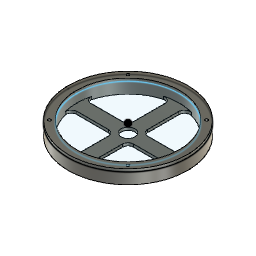
wing_interface_v1 (Autodesk Fusion 360 archive; units mm, degrees)
design "main_body_43mm_diameter"
Autodesk Fusion 360 part; units mm, degrees
(part 1 of 9)
sketch "Sketch1" plane through (0, 0, 0) normal (0, 0, 1) x (1, 0, 0)
  circle A0 centre (0, 0) radius 21.5
  circle A1 centre (0, 0) radius 18.5
  circle A2 centre (0, 0) radius 2.5
  line L0 (-2.5, 4.5) -> (-2.5, 15.8622)
  line L1 (2.5, 15.8622) -> (2.5, 4.5)
  line L2 (4.5, -2.5) -> (15.8806, -2.5)
  line L3 (15.8806, 2.5) -> (4.5, 2.5)
  line L4 (-2.5, -4.5) -> (-2.5, -15.8473)
  line L5 (2.5, -15.8473) -> (2.5, -4.5)
  line L6 (-4.5, -2.5) -> (-15.892, -2.5)
  line L7 (-15.9057, 2.5) -> (-4.5, 2.5)
  arc A3 (2.5, 4.5) -> (4.5, 2.5) centre (4.5, 4.5) ccw
  arc A4 (4.5, -2.5) -> (2.5, -4.5) centre (4.5, -4.5) ccw
  arc A5 (-2.5, -4.5) -> (-4.5, -2.5) centre (-4.5, -4.5) ccw
  arc A6 (-4.5, 2.5) -> (-2.5, 4.5) centre (-4.5, 4.5) ccw
  line L8 (-17.8692, 4.8804) -> (-17.9378, 4.526)
  line L9 (-17.8533, -4.8912) -> (-17.8867, -4.7239)
  arc A7 (-17.8692, 4.8804) -> (-15.9057, 2.5) centre (-15.9057, 4.5) ccw
  arc A8 (-15.892, -2.5) -> (-17.8533, -4.8912) centre (-15.892, -4.5) ccw
  line L10 (-4.926, -17.8014) -> (-5.3564, -17.7076)
  line L11 (4.926, -17.8014) -> (5.3564, -17.7076)
  arc A9 (-4.926, -17.8014) -> (-2.5, -15.8473) centre (-4.5, -15.8473) ccw
  arc A10 (2.5, -15.8473) -> (4.926, -17.8014) centre (4.5, -15.8473) ccw
  line L12 (17.8401, -4.9002) -> (17.8428, -4.8872)
  line L13 (17.8401, 4.9002) -> (17.8428, 4.8872)
  arc A11 (15.8806, 2.5) -> (17.8401, 4.9002) centre (15.8806, 4.5) ccw
  arc A12 (17.8401, -4.9002) -> (15.8806, -2.5) centre (15.8806, -4.5) ccw
  line L14 (4.9145, 17.8188) -> (5.1482, 17.7693)
  line L15 (-4.9145, 17.8188) -> (-5.1482, 17.7693)
  arc A13 (-2.5, 15.8622) -> (-4.9145, 17.8188) centre (-4.5, 15.8622) ccw
  arc A14 (4.9145, 17.8188) -> (2.5, 15.8622) centre (4.5, 15.8622) ccw
  dimension "d1" = 43
  dimension "d2" = 37
  dimension "d3" = 5
  dimension "d6" = 2
  dimension "d7" = 2
  dimension "d8" = 2
  dimension "d9" = 2
  dimension "d10" = 2
  dimension "d11" = 2
  dimension "d12" = 2
  dimension "d13" = 2
  dimension "d14" = 2
  dimension "d15" = 2
  dimension "d16" = 2
  dimension "d17" = 2
  constraint concentric A0 A1
  constraint concentric A1 A2
  constraint vertical L0
  constraint vertical L1
  constraint horizontal L2
  constraint horizontal L3
  constraint vertical L4
  constraint vertical L5
  constraint horizontal L6
  constraint horizontal L7
  constraint tangent L1 A3
  constraint tangent L3 A3
  constraint tangent L2 A4
  constraint tangent L5 A4
  constraint tangent L6 A5
  constraint tangent L4 A5
  constraint tangent L7 A6
  constraint tangent L0 A6
  constraint coincident A1 L8.end
  constraint coincident A1 L9.end
  constraint tangent L8 A7
  constraint tangent L7 A7
  constraint tangent L9 A8
  constraint tangent L6 A8
  constraint coincident A1 L10.end
  constraint coincident A1 L11.end
  constraint tangent L10 A9
  constraint tangent L4 A9
  constraint tangent L11 A10
  constraint tangent L5 A10
  constraint coincident A1 L12.end
  constraint coincident A1 L13.end
  constraint tangent L13 A11
  constraint tangent L3 A11
  constraint tangent L12 A12
  constraint tangent L2 A12
  constraint coincident A1 L14.end
  constraint coincident A1 L15.end
  constraint tangent L15 A13
  constraint tangent L0 A13
  constraint tangent L14 A14
  constraint tangent L1 A14
  measures "d1" diameter of A0
  measures "d2" diameter of A1
  measures "d3" diameter of A2
  measures "d6" radius of A3
  measures "d7" radius of A4
  measures "d8" radius of A5
  measures "d9" radius of A6
  measures "d10" radius of A7
  measures "d11" radius of A8
  measures "d12" radius of A9
  measures "d13" radius of A10
  measures "d14" radius of A11
  measures "d15" radius of A12
  measures "d16" radius of A13
  measures "d17" radius of A14
extrude "Extrude1" add sketch "Sketch1" along normal blind 1 contours A1 L0 L1 L2 L3 L4 L5 L6 L7 A3 A4 A5 A6 A7 A8 L10 L11 A9 A10 A11 A12 L14 L15 A13 A14
sketch "Sketch2" plane through (0, 0, 0) normal (0, 0, 1) x (1, 0, 0)
  circle A0 centre (0, 0) radius 21.5
  circle A1 centre (0, 0) radius 18.5
  line L0 (0, 0) -> (20, 0) construction
  circle A2 centre (-14.1421, 14.1421) radius 0.5
  circle A3 centre (14.1421, 14.1421) radius 0.5
  circle A4 centre (14.1421, -14.1421) radius 0.5
  circle A5 centre (-14.1421, -14.1421) radius 0.5
  dimension "d20" = 43
  dimension "d21" = 37
  dimension "d24" = 1
  dimension "d25" = 1
  dimension "d26" = 1
  dimension "d27" = 1
  constraint coincident A0.centre A1.centre
  constraint concentric A0 A1
  constraint horizontal L0
  measures "d20" diameter of A0
  measures "d21" diameter of A1
  measures "d24" diameter of A2
  measures "d25" diameter of A3
  measures "d26" diameter of A4
  measures "d27" diameter of A5
extrude "Extrude2" add sketch "Sketch2" along normal blind 4
sketch "Sketch3" plane through (0, 0, 4) normal (0, 0, 1) x (-1, 0, 0)
  circle A0 centre (-14.1421, 14.1421) radius 0.5
  circle A1 centre (14.1421, -14.1421) radius 0.5
  circle A2 centre (14.1421, 14.1421) radius 0.5
  circle A3 centre (-14.1421, -14.1421) radius 0.5
  circle A4 centre (0, 0) radius 18.5
  circle A5 centre (0, 0) radius 21.5
sketch "Sketch4" plane through (0, 0, 4) normal (0, 0, 1) x (-1, 0, 0)
  circle A0 centre (0, 0) radius 21.5
  circle A1 centre (0, 0) radius 18.5166
  dimension "d30" = 43
  constraint coincident A0.centre A1.centre
  constraint concentric A0 A1
  measures "d30" diameter of A0
extrude "Extrude3" add sketch "Sketch3" along normal blind 1

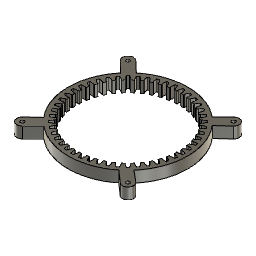
design "second_internal_gear_29mm_diameter"
Autodesk Fusion 360 part; units mm, degrees
sketch "Sketch1" plane through (0, 0, 0) normal (0, 0, 1) x (1, 0, 0)
  spline S0 degree 5 poles (13.9316, -0.5334) (13.9316, -0.5334) (13.9317, -0.5334) (13.9319, -0.5334) (13.9321, -0.5334) (13.9325, -0.5334) (13.9329, -0.5334) (13.9333, -0.5335) (13.9338, -0.5335) (13.9344, -0.5335) (13.935, -0.5335) (13.9356, -0.5335) (13.9364, -0.5335) (13.9371, -0.5335) (13.9379, -0.5335) (13.9388, -0.5335) (13.9397, -0.5335) (13.9406, -0.5335) (13.9416, -0.5335) (13.9427, -0.5335) (13.9438, -0.5335) (13.9449, -0.5335) (13.9461, -0.5335) (13.9473, -0.5335) (13.9486, -0.5335) (13.9499, -0.5335) (13.9513, -0.5335) (13.9527, -0.5334) (13.9542, -0.5334) (13.9557, -0.5334) (13.9572, -0.5333) (13.9588, -0.5333) (13.9605, -0.5333) (13.9621, -0.5332) (13.9639, -0.5332) (13.9656, -0.5331) (13.9674, -0.533) (13.9693, -0.533) (13.9712, -0.5329) (13.9731, -0.5328) (13.9751, -0.5328) (13.9771, -0.5327) (13.9792, -0.5326) (13.9813, -0.5325) (13.9834, -0.5324) (13.9856, -0.5323) (13.9878, -0.5322) (13.9901, -0.532) (13.9924, -0.5319) (13.9947, -0.5318) (13.9971, -0.5316) (13.9996, -0.5315) (14.002, -0.5313) (14.0045, -0.5312) (14.0071, -0.531) (14.0096, -0.5308) (14.0123, -0.5307) (14.0149, -0.5305) (14.0176, -0.5303) (14.0203, -0.5301) (14.0231, -0.5299) (14.0259, -0.5297) (14.0287, -0.5294) (14.0316, -0.5292) (14.0345, -0.529) (14.0375, -0.5287) (14.0405, -0.5284) (14.0435, -0.5282) (14.0466, -0.5279) (14.0497, -0.5276) (14.0528, -0.5273) (14.056, -0.527) (14.0592, -0.5267) (14.0624, -0.5264) (14.0657, -0.5261) (14.069, -0.5257) (14.0723, -0.5254) (14.0757, -0.525) (14.0791, -0.5247) (14.0825, -0.5243) (14.086, -0.5239) (14.0895, -0.5235) (14.0931, -0.5231) (14.0967, -0.5227) (14.1003, -0.5223) (14.1039, -0.5218) (14.1076, -0.5214) (14.1113, -0.5209) (14.115, -0.5205) (14.1188, -0.52) (14.1226, -0.5195) (14.1264, -0.519) (14.1303, -0.5185) (14.1342, -0.518) (14.1381, -0.5175) (14.1421, -0.5169) (14.1461, -0.5164) (14.1501, -0.5158) (14.1542, -0.5152) (14.1583, -0.5147) (14.1624, -0.5141) (14.1665, -0.5135) (14.1707, -0.5128) (14.1749, -0.5122) (14.1792, -0.5116) (14.1834, -0.5109) (14.1877, -0.5103) (14.1921, -0.5096) (14.1964, -0.5089) (14.2008, -0.5082) (14.2052, -0.5075) (14.2097, -0.5068) (14.2141, -0.506) (14.2186, -0.5053) (14.2232, -0.5045) (14.2277, -0.5037) (14.2323, -0.503) (14.2369, -0.5022) (14.2416, -0.5013) (14.2462, -0.5005) (14.2509, -0.4997) (14.2557, -0.4988) (14.2604, -0.498) (14.2652, -0.4971) (14.27, -0.4962) (14.2748, -0.4953) (14.2797, -0.4944) (14.2846, -0.4935) (14.2895, -0.4925) (14.2944, -0.4916) (14.2994, -0.4906) (14.3044, -0.4897) (14.3094, -0.4887) (14.3145, -0.4877) (14.3195, -0.4866) (14.3246, -0.4856) (14.3298, -0.4846) (14.3349, -0.4835) (14.3401, -0.4824) (14.3453, -0.4813) (14.3505, -0.4802) (14.3558, -0.4791) (14.361, -0.478) (14.3663, -0.4769) (14.3717, -0.4757) (14.377, -0.4745) (14.3824, -0.4734) (14.3878, -0.4722) (14.3932, -0.4709) (14.3987, -0.4697) (14.4041, -0.4685) (14.4096, -0.4672) (14.4152, -0.466) (14.4207, -0.4647) (14.4263, -0.4634) (14.4319, -0.4621) (14.4375, -0.4607) (14.4431, -0.4594) (14.4488, -0.458) (14.4545, -0.4567) (14.4602, -0.4553) (14.4659, -0.4539) (14.4717, -0.4525) (14.4774, -0.451) (14.4832, -0.4496) (14.4891, -0.4481) (14.4949, -0.4466) (14.5008, -0.4452) (14.5067, -0.4437) (14.5126, -0.4421) (14.5185, -0.4406) (14.5244, -0.439) (14.5304, -0.4375) (14.5364, -0.4359) (14.5424, -0.4343) (14.5485, -0.4327) (14.5545, -0.4311) (14.5606, -0.4294) (14.5667, -0.4278) (14.5729, -0.4261) (14.579, -0.4244) (14.5852, -0.4227) (14.5914, -0.421) (14.5976, -0.4192) (14.6038, -0.4175) (14.61, -0.4157) (14.6163, -0.4139) (14.6226, -0.4121) (14.6289, -0.4103) (14.6352, -0.4085) (14.6416, -0.4066) (14.648, -0.4048) (14.6544, -0.4029) (14.6608, -0.401) (14.6672, -0.3991) (14.6736, -0.3971) (14.6801, -0.3952) (14.6866, -0.3932) (14.6931, -0.3913) (14.6996, -0.3893) (14.7062, -0.3872) (14.7128, -0.3852) (14.7193, -0.3832) (14.7259, -0.3811) (14.7326, -0.379) (14.7392, -0.377) (14.7459, -0.3748) (14.7525, -0.3727) (14.7592, -0.3706) (14.7659, -0.3684) (14.7727, -0.3662) (14.7794, -0.3641) (14.7862, -0.3618) (14.793, -0.3596) (14.7998, -0.3574) (14.8066, -0.3551) (14.8134, -0.3528) (14.8203, -0.3506) (14.8272, -0.3482) (14.8341, -0.3459) (14.841, -0.3436) (14.8479, -0.3412) (14.8549, -0.3388) (14.8618, -0.3364) (14.8688, -0.334) (14.8758, -0.3316) (14.8828, -0.3292) (14.8898, -0.3267) (14.8969, -0.3242) (14.9039, -0.3217) (14.911, -0.3192) (14.9181, -0.3167) (14.9252, -0.3141) (14.9324, -0.3116) (14.9395, -0.309) (14.9467, -0.3064) (14.9538, -0.3038) (14.961, -0.3011) (14.9682, -0.2985) (14.9755, -0.2958) (14.9827, -0.2931) (14.9885, -0.291) (14.9929, -0.2893) (14.9958, -0.2883) (14.9972, -0.2877) knots 0 0 0 0 0 0 0.00416667 0.00833333 0.0125 0.01666667 0.02083333 0.025 0.02916667 0.03333333 0.0375 0.04166667 0.04583333 0.05 0.05416667 0.05833333 0.0625 0.06666667 0.07083333 0.075 0.07916667 0.08333333 0.0875 0.09166667 0.09583333 0.1 0.10416667 0.10833333 0.1125 0.11666667 0.12083333 0.125 0.12916667 0.13333333 0.1375 0.14166667 0.14583333 0.15 0.15416667 0.15833333 0.1625 0.16666667 0.17083333 0.175 0.17916667 0.18333333 0.1875 0.19166667 0.19583333 0.2 0.20416667 0.20833333 0.2125 0.21666667 0.22083333 0.225 0.22916667 0.23333333 0.2375 0.24166667 0.24583333 0.25 0.25416667 0.25833333 0.2625 0.26666667 0.27083333 0.275 0.27916667 0.28333333 0.2875 0.29166667 0.29583333 0.3 0.30416667 0.30833333 0.3125 0.31666667 0.32083333 0.325 0.32916667 0.33333333 0.3375 0.34166667 0.34583333 0.35 0.35416667 0.35833333 0.3625 0.36666667 0.37083333 0.375 0.37916667 0.38333333 0.3875 0.39166667 0.39583333 0.4 0.40416667 0.40833333 0.4125 0.41666667 0.42083333 0.425 0.42916667 0.43333333 0.4375 0.44166667 0.44583333 0.45 0.45416667 0.45833333 0.4625 0.46666667 0.47083333 0.475 0.47916667 0.48333333 0.4875 0.49166667 0.49583333 0.5 0.50416667 0.50833333 0.5125 0.51666667 0.52083333 0.525 0.52916667 0.53333333 0.5375 0.54166667 0.54583333 0.55 0.55416667 0.55833333 0.5625 0.56666667 0.57083333 0.575 0.57916667 0.58333333 0.5875 0.59166667 0.59583333 0.6 0.60416667 0.60833333 0.6125 0.61666667 0.62083333 0.625 0.62916667 0.63333333 0.6375 0.64166667 0.64583333 0.65 0.65416667 0.65833333 0.6625 0.66666667 0.67083333 0.675 0.67916667 0.68333333 0.6875 0.69166667 0.69583333 0.7 0.70416667 0.70833333 0.7125 0.71666667 0.72083333 0.725 0.72916667 0.73333333 0.7375 0.74166667 0.74583333 0.75 0.75416667 0.75833333 0.7625 0.76666667 0.77083333 0.775 0.77916667 0.78333333 0.7875 0.79166667 0.79583333 0.8 0.80416667 0.80833333 0.8125 0.81666667 0.82083333 0.825 0.82916667 0.83333333 0.8375 0.84166667 0.84583333 0.85 0.85416667 0.85833333 0.8625 0.86666667 0.87083333 0.875 0.87916667 0.88333333 0.8875 0.89166667 0.89583333 0.9 0.90416667 0.90833333 0.9125 0.91666667 0.92083333 0.925 0.92916667 0.93333333 0.9375 0.94166667 0.94583333 0.95 0.95416667 0.95833333 0.9625 0.96666667 0.97083333 0.975 0.97916667 0.98333333 0.9875 0.99166667 0.99583333 1 1 1 1 1 1
  spline S1 degree 5 poles (13.9316, 0.5334) (13.9316, 0.5334) (13.9317, 0.5334) (13.9319, 0.5334) (13.9321, 0.5334) (13.9325, 0.5334) (13.9329, 0.5334) (13.9333, 0.5335) (13.9338, 0.5335) (13.9344, 0.5335) (13.935, 0.5335) (13.9356, 0.5335) (13.9364, 0.5335) (13.9371, 0.5335) (13.9379, 0.5335) (13.9388, 0.5335) (13.9397, 0.5335) (13.9406, 0.5335) (13.9416, 0.5335) (13.9427, 0.5335) (13.9438, 0.5335) (13.9449, 0.5335) (13.9461, 0.5335) (13.9473, 0.5335) (13.9486, 0.5335) (13.9499, 0.5335) (13.9513, 0.5335) (13.9527, 0.5334) (13.9542, 0.5334) (13.9557, 0.5334) (13.9572, 0.5333) (13.9588, 0.5333) (13.9605, 0.5333) (13.9621, 0.5332) (13.9639, 0.5332) (13.9656, 0.5331) (13.9674, 0.533) (13.9693, 0.533) (13.9712, 0.5329) (13.9731, 0.5328) (13.9751, 0.5328) (13.9771, 0.5327) (13.9792, 0.5326) (13.9813, 0.5325) (13.9834, 0.5324) (13.9856, 0.5323) (13.9878, 0.5322) (13.9901, 0.532) (13.9924, 0.5319) (13.9947, 0.5318) (13.9971, 0.5316) (13.9996, 0.5315) (14.002, 0.5313) (14.0045, 0.5312) (14.0071, 0.531) (14.0096, 0.5308) (14.0123, 0.5307) (14.0149, 0.5305) (14.0176, 0.5303) (14.0203, 0.5301) (14.0231, 0.5299) (14.0259, 0.5297) (14.0287, 0.5294) (14.0316, 0.5292) (14.0345, 0.529) (14.0375, 0.5287) (14.0405, 0.5284) (14.0435, 0.5282) (14.0466, 0.5279) (14.0497, 0.5276) (14.0528, 0.5273) (14.056, 0.527) (14.0592, 0.5267) (14.0624, 0.5264) (14.0657, 0.5261) (14.069, 0.5257) (14.0723, 0.5254) (14.0757, 0.525) (14.0791, 0.5247) (14.0825, 0.5243) (14.086, 0.5239) (14.0895, 0.5235) (14.0931, 0.5231) (14.0967, 0.5227) (14.1003, 0.5223) (14.1039, 0.5218) (14.1076, 0.5214) (14.1113, 0.5209) (14.115, 0.5205) (14.1188, 0.52) (14.1226, 0.5195) (14.1264, 0.519) (14.1303, 0.5185) (14.1342, 0.518) (14.1381, 0.5175) (14.1421, 0.5169) (14.1461, 0.5164) (14.1501, 0.5158) (14.1542, 0.5152) (14.1583, 0.5147) (14.1624, 0.5141) (14.1665, 0.5135) (14.1707, 0.5128) (14.1749, 0.5122) (14.1792, 0.5116) (14.1834, 0.5109) (14.1877, 0.5103) (14.1921, 0.5096) (14.1964, 0.5089) (14.2008, 0.5082) (14.2052, 0.5075) (14.2097, 0.5068) (14.2141, 0.506) (14.2186, 0.5053) (14.2232, 0.5045) (14.2277, 0.5037) (14.2323, 0.503) (14.2369, 0.5022) (14.2416, 0.5013) (14.2462, 0.5005) (14.2509, 0.4997) (14.2557, 0.4988) (14.2604, 0.498) (14.2652, 0.4971) (14.27, 0.4962) (14.2748, 0.4953) (14.2797, 0.4944) (14.2846, 0.4935) (14.2895, 0.4925) (14.2944, 0.4916) (14.2994, 0.4906) (14.3044, 0.4897) (14.3094, 0.4887) (14.3145, 0.4877) (14.3195, 0.4866) (14.3246, 0.4856) (14.3298, 0.4846) (14.3349, 0.4835) (14.3401, 0.4824) (14.3453, 0.4813) (14.3505, 0.4802) (14.3558, 0.4791) (14.361, 0.478) (14.3663, 0.4769) (14.3717, 0.4757) (14.377, 0.4745) (14.3824, 0.4734) (14.3878, 0.4722) (14.3932, 0.4709) (14.3987, 0.4697) (14.4041, 0.4685) (14.4096, 0.4672) (14.4152, 0.466) (14.4207, 0.4647) (14.4263, 0.4634) (14.4319, 0.4621) (14.4375, 0.4607) (14.4431, 0.4594) (14.4488, 0.458) (14.4545, 0.4567) (14.4602, 0.4553) (14.4659, 0.4539) (14.4717, 0.4525) (14.4774, 0.451) (14.4832, 0.4496) (14.4891, 0.4481) (14.4949, 0.4466) (14.5008, 0.4452) (14.5067, 0.4437) (14.5126, 0.4421) (14.5185, 0.4406) (14.5244, 0.439) (14.5304, 0.4375) (14.5364, 0.4359) (14.5424, 0.4343) (14.5485, 0.4327) (14.5545, 0.4311) (14.5606, 0.4294) (14.5667, 0.4278) (14.5729, 0.4261) (14.579, 0.4244) (14.5852, 0.4227) (14.5914, 0.421) (14.5976, 0.4192) (14.6038, 0.4175) (14.61, 0.4157) (14.6163, 0.4139) (14.6226, 0.4121) (14.6289, 0.4103) (14.6352, 0.4085) (14.6416, 0.4066) (14.648, 0.4048) (14.6544, 0.4029) (14.6608, 0.401) (14.6672, 0.3991) (14.6736, 0.3971) (14.6801, 0.3952) (14.6866, 0.3932) (14.6931, 0.3913) (14.6996, 0.3893) (14.7062, 0.3872) (14.7128, 0.3852) (14.7193, 0.3832) (14.7259, 0.3811) (14.7326, 0.379) (14.7392, 0.377) (14.7459, 0.3748) (14.7525, 0.3727) (14.7592, 0.3706) (14.7659, 0.3684) (14.7727, 0.3662) (14.7794, 0.3641) (14.7862, 0.3618) (14.793, 0.3596) (14.7998, 0.3574) (14.8066, 0.3551) (14.8134, 0.3528) (14.8203, 0.3506) (14.8272, 0.3482) (14.8341, 0.3459) (14.841, 0.3436) (14.8479, 0.3412) (14.8549, 0.3388) (14.8618, 0.3364) (14.8688, 0.334) (14.8758, 0.3316) (14.8828, 0.3292) (14.8898, 0.3267) (14.8969, 0.3242) (14.9039, 0.3217) (14.911, 0.3192) (14.9181, 0.3167) (14.9252, 0.3141) (14.9324, 0.3116) (14.9395, 0.309) (14.9467, 0.3064) (14.9538, 0.3038) (14.961, 0.3011) (14.9682, 0.2985) (14.9755, 0.2958) (14.9827, 0.2931) (14.9885, 0.291) (14.9929, 0.2893) (14.9958, 0.2883) (14.9972, 0.2877) knots 0 0 0 0 0 0 0.00416667 0.00833333 0.0125 0.01666667 0.02083333 0.025 0.02916667 0.03333333 0.0375 0.04166667 0.04583333 0.05 0.05416667 0.05833333 0.0625 0.06666667 0.07083333 0.075 0.07916667 0.08333333 0.0875 0.09166667 0.09583333 0.1 0.10416667 0.10833333 0.1125 0.11666667 0.12083333 0.125 0.12916667 0.13333333 0.1375 0.14166667 0.14583333 0.15 0.15416667 0.15833333 0.1625 0.16666667 0.17083333 0.175 0.17916667 0.18333333 0.1875 0.19166667 0.19583333 0.2 0.20416667 0.20833333 0.2125 0.21666667 0.22083333 0.225 0.22916667 0.23333333 0.2375 0.24166667 0.24583333 0.25 0.25416667 0.25833333 0.2625 0.26666667 0.27083333 0.275 0.27916667 0.28333333 0.2875 0.29166667 0.29583333 0.3 0.30416667 0.30833333 0.3125 0.31666667 0.32083333 0.325 0.32916667 0.33333333 0.3375 0.34166667 0.34583333 0.35 0.35416667 0.35833333 0.3625 0.36666667 0.37083333 0.375 0.37916667 0.38333333 0.3875 0.39166667 0.39583333 0.4 0.40416667 0.40833333 0.4125 0.41666667 0.42083333 0.425 0.42916667 0.43333333 0.4375 0.44166667 0.44583333 0.45 0.45416667 0.45833333 0.4625 0.46666667 0.47083333 0.475 0.47916667 0.48333333 0.4875 0.49166667 0.49583333 0.5 0.50416667 0.50833333 0.5125 0.51666667 0.52083333 0.525 0.52916667 0.53333333 0.5375 0.54166667 0.54583333 0.55 0.55416667 0.55833333 0.5625 0.56666667 0.57083333 0.575 0.57916667 0.58333333 0.5875 0.59166667 0.59583333 0.6 0.60416667 0.60833333 0.6125 0.61666667 0.62083333 0.625 0.62916667 0.63333333 0.6375 0.64166667 0.64583333 0.65 0.65416667 0.65833333 0.6625 0.66666667 0.67083333 0.675 0.67916667 0.68333333 0.6875 0.69166667 0.69583333 0.7 0.70416667 0.70833333 0.7125 0.71666667 0.72083333 0.725 0.72916667 0.73333333 0.7375 0.74166667 0.74583333 0.75 0.75416667 0.75833333 0.7625 0.76666667 0.77083333 0.775 0.77916667 0.78333333 0.7875 0.79166667 0.79583333 0.8 0.80416667 0.80833333 0.8125 0.81666667 0.82083333 0.825 0.82916667 0.83333333 0.8375 0.84166667 0.84583333 0.85 0.85416667 0.85833333 0.8625 0.86666667 0.87083333 0.875 0.87916667 0.88333333 0.8875 0.89166667 0.89583333 0.9 0.90416667 0.90833333 0.9125 0.91666667 0.92083333 0.925 0.92916667 0.93333333 0.9375 0.94166667 0.94583333 0.95 0.95416667 0.95833333 0.9625 0.96666667 0.97083333 0.975 0.97916667 0.98333333 0.9875 0.99166667 0.99583333 1 1 1 1 1 1
  spline S2 degree 5 poles (13.9311, -0.5334) (13.9311, -0.5334) (13.9312, -0.5334) (13.9312, -0.5334) (13.9313, -0.5334) (13.9314, -0.5334) (13.9315, -0.5334) (13.9315, -0.5334) (13.9316, -0.5334) (13.9316, -0.5334) knots 0 0 0 0 0 0 0.2 0.4 0.6 0.8 1 1 1 1 1 1
  spline S3 degree 5 poles (13.9311, 0.5334) (13.9311, 0.5334) (13.9312, 0.5334) (13.9312, 0.5334) (13.9313, 0.5334) (13.9314, 0.5334) (13.9315, 0.5334) (13.9315, 0.5334) (13.9316, 0.5334) (13.9316, 0.5334) knots 0 0 0 0 0 0 0.2 0.4 0.6 0.8 1 1 1 1 1 1
  line L0 (0, 0) -> (13.9311, -0.5334)
  line L1 (0, 0) -> (13.9311, 0.5334)
  arc A0 (14.9972, -0.2877) -> (14.9972, 0.2877) centre (0, 0) ccw
  point P0 (13.9329, -0.5335)
  point P1 (13.9352, -0.5335)
  point P2 (13.9384, -0.5335)
  point P3 (13.9426, -0.5335)
  point P4 (13.9476, -0.5335)
  point P5 (13.9535, -0.5334)
  point P6 (13.9604, -0.5333)
  point P7 (13.9682, -0.533)
  point P8 (13.9769, -0.5327)
  point P9 (13.9865, -0.5322)
  point P10 (13.997, -0.5317)
  point P11 (14.0084, -0.5309)
  point P12 (14.0207, -0.5301)
  point P13 (14.034, -0.529)
  point P14 (14.0481, -0.5278)
  point P15 (14.0631, -0.5263)
  point P16 (14.0791, -0.5247)
  point P17 (14.0959, -0.5228)
  point P18 (14.1136, -0.5206)
  point P19 (14.1322, -0.5183)
  point P20 (14.1517, -0.5156)
  point P21 (14.1721, -0.5126)
  point P22 (14.1934, -0.5094)
  point P23 (14.2155, -0.5058)
  point P24 (14.2385, -0.5019)
  point P25 (14.2624, -0.4976)
  point P26 (14.2871, -0.493)
  point P27 (14.3127, -0.488)
  point P28 (14.3392, -0.4826)
  point P29 (14.3665, -0.4768)
  point P30 (14.3947, -0.4706)
  point P31 (14.4237, -0.464)
  point P32 (14.4535, -0.4569)
  point P33 (14.4842, -0.4493)
  point P34 (14.5157, -0.4413)
  point P35 (14.548, -0.4328)
  point P36 (14.5811, -0.4238)
  point P37 (14.615, -0.4143)
  point P38 (14.6497, -0.4042)
  point P39 (14.6853, -0.3936)
  point P40 (14.7216, -0.3825)
  point P41 (14.7587, -0.3708)
  point P42 (14.7965, -0.3584)
  point P43 (14.8352, -0.3455)
  point P44 (14.8746, -0.332)
  point P45 (14.9147, -0.3179)
  point P46 (14.9556, -0.3031)
  point P47 (13.9329, 0.5335)
  point P48 (13.9352, 0.5335)
  point P49 (13.9384, 0.5335)
  point P50 (13.9426, 0.5335)
  point P51 (13.9476, 0.5335)
  point P52 (13.9535, 0.5334)
  point P53 (13.9604, 0.5333)
  point P54 (13.9682, 0.533)
  point P55 (13.9769, 0.5327)
  point P56 (13.9865, 0.5322)
  point P57 (13.997, 0.5317)
  point P58 (14.0084, 0.5309)
  point P59 (14.0207, 0.5301)
  point P60 (14.034, 0.529)
  point P61 (14.0481, 0.5278)
  point P62 (14.0631, 0.5263)
  point P63 (14.0791, 0.5247)
  point P64 (14.0959, 0.5228)
  point P65 (14.1136, 0.5206)
  point P66 (14.1322, 0.5183)
  point P67 (14.1517, 0.5156)
  point P68 (14.1721, 0.5126)
  point P69 (14.1934, 0.5094)
  point P70 (14.2155, 0.5058)
  point P71 (14.2385, 0.5019)
  point P72 (14.2624, 0.4976)
  point P73 (14.2871, 0.493)
  point P74 (14.3127, 0.488)
  point P75 (14.3392, 0.4826)
  point P76 (14.3665, 0.4768)
  point P77 (14.3947, 0.4706)
  point P78 (14.4237, 0.464)
  point P79 (14.4535, 0.4569)
  point P80 (14.4842, 0.4493)
  point P81 (14.5157, 0.4413)
  point P82 (14.548, 0.4328)
  point P83 (14.5811, 0.4238)
  point P84 (14.615, 0.4143)
  point P85 (14.6497, 0.4042)
  point P86 (14.6853, 0.3936)
  point P87 (14.7216, 0.3825)
  point P88 (14.7587, 0.3708)
  point P89 (14.7965, 0.3584)
  point P90 (14.8352, 0.3455)
  point P91 (14.8746, 0.332)
  point P92 (14.9147, 0.3179)
  point P93 (14.9556, 0.3031)
sketch "Sketch2" plane through (0, 0, 0) normal (0, 0, 1) x (1, 0, 0)
  circle A0 centre (0, 0) radius 16
  circle A1 centre (0, 0) radius 13.65
  circle A2 centre (0, 0) radius 13.65
extrude "Extrude1" add sketch "Sketch2" along normal blind 3
extrude "Extrude2" cut sketch "Sketch1" along normal blind 3
pattern_circular "C-Pattern1" count 48 over 360 about axis through (0, 0, 1.75) along (0, 0, 1) of "Extrude2"
sketch "Sketch3" plane through (0, 0, 0) normal (0, 0, 1) x (1, 0, 0)
  line L0 (0, 0) -> (48.7031, 0) construction
  line L1 (48.7031, 0) -> (48.7031, 3) construction
  line L2 (48.7031, 3) -> (0, 3) construction
  line L3 (0, 3) -> (0, 0) construction
  constraint perpendicular L0 L1
  constraint parallel L0 L2
  constraint parallel L1 L3
sketch "Sketch4" plane through (0, 0, 0) normal (0, 0, 1) x (1, 0, 0)
  line L0 (0, 0) -> (20, 0) construction
  circle A0 centre (14.1421, 14.1421) radius 0.5
  circle A1 centre (14.1421, -14.1421) radius 0.5
  circle A2 centre (-14.1421, -14.1421) radius 0.5
  circle A3 centre (-14.1421, 14.1421) radius 0.5
  line L1 (15.1511, 13.0322) -> (11.8585, 10.0393)
  line L2 (11.8585, 10.0393) -> (11, 11)
  line L3 (13.0755, 15.1968) -> (9.9303, 12.0161)
  line L4 (9.9303, 12.0161) -> (11, 11)
  arc A4 (15.1511, 13.0322) -> (13.0755, 15.1968) centre (14.1421, 14.1421) ccw
  line L5 (15.1839, -13.0629) -> (11.5, -10)
  line L6 (13.342, -15.4109) -> (9.5, -12)
  line L7 (9.5, -12) -> (11.5, -10)
  arc A5 (12.9771, -15.087) -> (15.013, -12.9208) centre (14.1421, -14.1421) ccw
  line L8 (-11, -11) -> (-10, -12)
  line L9 (-13.0815, -15.2028) -> (-9.9338, -12.0551)
  line L10 (-9.9338, -12.0551) -> (-10, -12)
  line L11 (-15.2028, -13.0815) -> (-12, -10.1)
  line L12 (-12, -10.1) -> (-11, -11)
  arc A6 (-15.1243, -13.0084) -> (-13.0815, -15.2028) centre (-14.1421, -14.1421) ccw
  line L13 (-15.1805, 13.0596) -> (-11.7229, 9.7707)
  line L14 (-13.0948, 15.216) -> (-9.7671, 11.9704)
  line L15 (-9.7671, 11.9704) -> (-11.7229, 9.7707)
  arc A7 (-13.0948, 15.216) -> (-15.1714, 13.051) centre (-14.1421, 14.1421) ccw
  dimension "d11" = 1
  dimension "d12" = 1
  dimension "d13" = 1
  dimension "d14" = 1
  dimension "d15" = 3
  dimension "d16" = 3
  dimension "d17" = 3
  dimension "d18" = 3
  constraint horizontal L0
  constraint coincident L0.start origin
  constraint concentric A0 A4
  constraint tangent L1 A4
  constraint tangent L3 A4
  constraint concentric A1 A5
  constraint coincident L5.start A5
  constraint coincident L6.start A5
  constraint coincident L6 A5.start
  constraint coincident L5 A5.end
  constraint concentric A2 A6
  constraint tangent L9 A6
  constraint coincident L11.start A6
  constraint coincident L11 A6.start
  constraint concentric A3 A7
  constraint coincident L13.start A7
  constraint tangent L14 A7
  constraint coincident L13 A7.end
  measures "d11" diameter of A0
  measures "d12" diameter of A1
  measures "d13" diameter of A2
  measures "d14" diameter of A3
  measures "d15" diameter of A4
  measures "d16" diameter of A5
  measures "d17" diameter of A6
  measures "d18" diameter of A7
extrude "Extrude3" add sketch "Sketch4" along normal blind 3 contours L1 L2 L3 L4 A4 | L5 L6 L7 A5 | L8 L9 L10 L11 L12 A6 | L13 L14 L15 A7

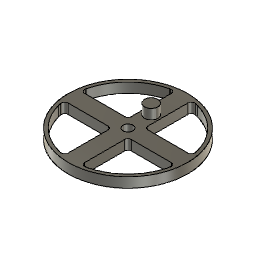
design "spinning_part_36mm_diameter"
Autodesk Fusion 360 part; units mm, degrees
sketch "Sketch1" plane through (0, 0, 0) normal (0, 0, 1) x (1, 0, 0)
  circle A0 centre (0, 0) radius 18
  line L0 (-2.5, 3.5) -> (-2.5, 15.5984)
  line L1 (2.5, 15.5848) -> (2.5, 3.5)
  line L2 (3.5, 2.5) -> (15.5763, 2.5)
  line L3 (17.3145, 2.5) -> (17.3145, -2.5)
  line L4 (15.5763, -2.5) -> (3.5, -2.5)
  line L5 (-3.5, -2.5) -> (-15.5736, -2.5)
  line L6 (-15.5966, 2.5) -> (-3.5, 2.5)
  line L7 (2.5, -3.5) -> (2.5, -15.5822)
  line L8 (-2.5, -15.565) -> (-2.5, -3.5)
  arc A1 (3.5, -2.5) -> (2.5, -3.5) centre (3.5, -3.5) ccw
  arc A2 (-2.5, -3.5) -> (-3.5, -2.5) centre (-3.5, -3.5) ccw
  arc A3 (2.5, 3.5) -> (3.5, 2.5) centre (3.5, 3.5) ccw
  arc A4 (-3.5, 2.5) -> (-2.5, 3.5) centre (-3.5, 3.5) ccw
  line L9 (3.7044, 16.5636) -> (4.4389, 16.4103)
  line L10 (-3.6937, 16.5794) -> (-4.0793, 16.5033)
  arc A5 (-2.5, 15.5984) -> (-3.6937, 16.5794) centre (-3.5, 15.5984) ccw
  arc A6 (3.7044, 16.5636) -> (2.5, 15.5848) centre (3.5, 15.5848) ccw
  line L11 (16.5538, 3.711) -> (16.3494, 4.6582)
  line L12 (16.5538, -3.711) -> (16.3494, -4.6582)
  arc A7 (15.5763, 2.5) -> (16.5538, 3.711) centre (15.5763, 3.5) ccw
  arc A8 (16.5538, -3.711) -> (15.5763, -2.5) centre (15.5763, -3.5) ccw
  line L13 (3.7064, -16.5606) -> (4.506, -16.3919)
  line L14 (-3.7196, -16.5406) -> (-4.9466, -16.2644)
  arc A9 (-3.7196, -16.5406) -> (-2.5, -15.565) centre (-3.5, -15.565) ccw
  arc A10 (2.5, -15.5822) -> (3.7064, -16.5606) centre (3.5, -15.5822) ccw
  line L15 (-16.5774, 3.6951) -> (-16.4916, 4.1264)
  line L16 (-16.5507, -3.713) -> (-16.3296, -4.7268)
  arc A11 (-16.5774, 3.6951) -> (-15.5966, 2.5) centre (-15.5966, 3.5) ccw
  arc A12 (-15.5736, -2.5) -> (-16.5507, -3.713) centre (-15.5736, -3.5) ccw
  arc A13 (-16.3296, -4.7268) -> (-4.9466, -16.2644) centre (0, 0) ccw
  arc A14 (4.506, -16.3919) -> (16.3494, -4.6582) centre (0, 0) ccw
  arc A15 (16.3494, 4.6582) -> (4.4389, 16.4103) centre (0, 0) ccw
  arc A16 (-4.0793, 16.5033) -> (-16.4916, 4.1264) centre (0, 0) ccw
  circle A17 centre (0, 0) radius 1.5
  dimension "d1" = 34
  dimension "d2" = 36
  dimension "d7" = 1
  dimension "d8" = 1
  dimension "d9" = 1
  dimension "d10" = 1
  dimension "d11" = 1
  dimension "d12" = 1
  dimension "d13" = 1
  dimension "d14" = 1
  dimension "d15" = 1
  dimension "d16" = 1
  dimension "d17" = 1
  dimension "d18" = 1
  dimension "d19" = 3
  constraint vertical L0
  constraint vertical L1
  constraint horizontal L2
  constraint vertical L3
  constraint horizontal L4
  constraint horizontal L5
  constraint horizontal L6
  constraint vertical L7
  constraint vertical L8
  constraint tangent L7 A1
  constraint tangent L4 A1
  constraint tangent L5 A2
  constraint tangent L8 A2
  constraint tangent L1 A3
  constraint tangent L2 A3
  constraint tangent L6 A4
  constraint tangent L0 A4
  constraint coincident L9.end A13
  constraint coincident L10.end A13
  constraint tangent L10 A5
  constraint tangent L0 A5
  constraint tangent L9 A6
  constraint tangent L1 A6
  constraint coincident L11.end A13
  constraint coincident L12.end A13
  constraint coincident L3.start L2
  constraint tangent L11 A7
  constraint tangent L2 A7
  constraint coincident L3.end L4
  constraint tangent L4 A8
  constraint tangent L12 A8
  constraint coincident L13.end A13
  constraint tangent L14 A9
  constraint tangent L8 A9
  constraint tangent L13 A10
  constraint tangent L7 A10
  constraint tangent L15 A11
  constraint tangent L6 A11
  constraint tangent L16 A12
  constraint tangent L5 A12
  constraint concentric A13 A14
  constraint concentric A14 A15
  constraint concentric A15 A16
  constraint concentric A14 A17
  measures "d1" diameter of A13
  measures "d2" diameter of A0
  measures "d7" radius of A1
  measures "d8" radius of A2
  measures "d9" radius of A3
  measures "d10" radius of A4
  measures "d11" radius of A5
  measures "d12" radius of A6
  measures "d13" radius of A7
  measures "d14" radius of A8
  measures "d15" radius of A9
  measures "d16" radius of A10
  measures "d17" radius of A11
  measures "d18" radius of A12
  measures "d19" diameter of A17
extrude "Extrude1" add sketch "Sketch1" along normal blind 3
sketch "Sketch2" plane through (0, 0, 3) normal (0, 0, 1) x (-1, 0, 0)
  arc A0 (-16.5538, 3.711) -> (-15.5763, 2.5) centre (-15.5763, 3.5) ccw
  line L0 (-16.5538, 3.711) -> (-16.3494, 4.6582)
  arc A1 (-4.506, 16.3919) -> (-16.3494, 4.6582) centre (0, 0) ccw
  line L1 (-4.506, 16.3919) -> (-3.7064, 16.5606)
  arc A2 (-2.5, 15.5822) -> (-3.7064, 16.5606) centre (-3.5, 15.5822) ccw
  line L2 (-2.5, 15.5822) -> (-2.5, 3.5)
  arc A3 (-3.5, 2.5) -> (-2.5, 3.5) centre (-3.5, 3.5) ccw
  line L3 (-3.5, 2.5) -> (-15.5763, 2.5)
  circle A4 centre (0, 0) radius 1.5
  arc A5 (16.5774, -3.6951) -> (15.5966, -2.5) centre (15.5966, -3.5) ccw
  line L4 (16.5774, -3.6951) -> (16.4916, -4.1264)
  arc A6 (4.0793, -16.5033) -> (16.4916, -4.1264) centre (0, 0) ccw
  line L5 (4.0793, -16.5033) -> (3.6937, -16.5794)
  arc A7 (2.5, -15.5984) -> (3.6937, -16.5794) centre (3.5, -15.5984) ccw
  line L6 (2.5, -15.5984) -> (2.5, -3.5)
  arc A8 (3.5, -2.5) -> (2.5, -3.5) centre (3.5, -3.5) ccw
  line L7 (3.5, -2.5) -> (15.5966, -2.5)
  arc A9 (-3.7044, -16.5636) -> (-2.5, -15.5848) centre (-3.5, -15.5848) ccw
  line L8 (-3.7044, -16.5636) -> (-4.4389, -16.4103)
  arc A10 (-16.3494, -4.6582) -> (-4.4389, -16.4103) centre (0, 0) ccw
  line L9 (-16.3494, -4.6582) -> (-16.5538, -3.711)
  arc A11 (-15.5763, -2.5) -> (-16.5538, -3.711) centre (-15.5763, -3.5) ccw
  line L10 (-15.5763, -2.5) -> (-3.5, -2.5)
  arc A12 (-2.5, -3.5) -> (-3.5, -2.5) centre (-3.5, -3.5) ccw
  line L11 (-2.5, -3.5) -> (-2.5, -15.5848)
  arc A13 (3.7196, 16.5406) -> (2.5, 15.565) centre (3.5, 15.565) ccw
  line L12 (3.7196, 16.5406) -> (4.9466, 16.2644)
  arc A14 (16.3296, 4.7268) -> (4.9466, 16.2644) centre (0, 0) ccw
  line L13 (16.3296, 4.7268) -> (16.5507, 3.713)
  arc A15 (15.5736, 2.5) -> (16.5507, 3.713) centre (15.5736, 3.5) ccw
  line L14 (15.5736, 2.5) -> (3.5, 2.5)
  arc A16 (2.5, 3.5) -> (3.5, 2.5) centre (3.5, 3.5) ccw
  line L15 (2.5, 3.5) -> (2.5, 15.565)
  circle A17 centre (0, 0) radius 18
  circle A18 centre (0, -7) radius 2
  dimension "d23" = 4
  measures "d23" diameter of A18
extrude "Extrude2" add sketch "Sketch2" along normal blind 3 contours A18

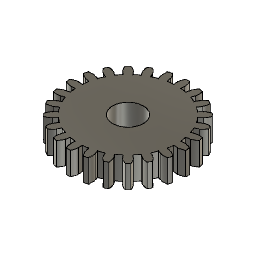
design "small_gear_15.591mm_diameter"
Autodesk Fusion 360 part; units mm, degrees
sketch "Sketch1" plane through (0, 0, 0) normal (0, 0, 1) x (1, 0, 0)
  spline S0 degree 5 poles (6.9535, -0.4945) (6.9535, -0.4945) (6.9536, -0.4945) (6.9537, -0.4945) (6.9539, -0.4945) (6.9541, -0.4945) (6.9545, -0.4945) (6.9548, -0.4946) (6.9552, -0.4946) (6.9556, -0.4946) (6.9561, -0.4946) (6.9566, -0.4946) (6.9571, -0.4947) (6.9577, -0.4947) (6.9583, -0.4947) (6.959, -0.4947) (6.9597, -0.4947) (6.9604, -0.4948) (6.9611, -0.4948) (6.9619, -0.4948) (6.9628, -0.4948) (6.9636, -0.4948) (6.9646, -0.4948) (6.9655, -0.4949) (6.9665, -0.4949) (6.9675, -0.4949) (6.9685, -0.4949) (6.9696, -0.4949) (6.9707, -0.4949) (6.9719, -0.4949) (6.9731, -0.4949) (6.9743, -0.4949) (6.9756, -0.4949) (6.9769, -0.4948) (6.9782, -0.4948) (6.9796, -0.4948) (6.9809, -0.4948) (6.9824, -0.4948) (6.9838, -0.4947) (6.9853, -0.4947) (6.9869, -0.4946) (6.9884, -0.4946) (6.99, -0.4946) (6.9916, -0.4945) (6.9933, -0.4944) (6.995, -0.4944) (6.9967, -0.4943) (6.9985, -0.4942) (7.0002, -0.4942) (7.0021, -0.4941) (7.0039, -0.494) (7.0058, -0.4939) (7.0077, -0.4938) (7.0096, -0.4937) (7.0116, -0.4936) (7.0136, -0.4934) (7.0156, -0.4933) (7.0177, -0.4932) (7.0198, -0.493) (7.0219, -0.4929) (7.0241, -0.4927) (7.0263, -0.4926) (7.0285, -0.4924) (7.0307, -0.4922) (7.033, -0.4921) (7.0353, -0.4919) (7.0376, -0.4917) (7.04, -0.4915) (7.0424, -0.4913) (7.0448, -0.4911) (7.0472, -0.4908) (7.0497, -0.4906) (7.0522, -0.4903) (7.0548, -0.4901) (7.0573, -0.4898) (7.0599, -0.4896) (7.0625, -0.4893) (7.0652, -0.489) (7.0678, -0.4887) (7.0705, -0.4884) (7.0733, -0.4881) (7.076, -0.4878) (7.0788, -0.4874) (7.0816, -0.4871) (7.0844, -0.4868) (7.0873, -0.4864) (7.0902, -0.486) (7.0931, -0.4857) (7.096, -0.4853) (7.099, -0.4849) (7.102, -0.4845) (7.105, -0.4841) (7.1081, -0.4836) (7.1111, -0.4832) (7.1142, -0.4827) (7.1173, -0.4823) (7.1205, -0.4818) (7.1237, -0.4813) (7.1268, -0.4809) (7.1301, -0.4804) (7.1333, -0.4798) (7.1366, -0.4793) (7.1399, -0.4788) (7.1432, -0.4782) (7.1465, -0.4777) (7.1499, -0.4771) (7.1533, -0.4766) (7.1567, -0.476) (7.1602, -0.4754) (7.1636, -0.4748) (7.1671, -0.4741) (7.1706, -0.4735) (7.1741, -0.4729) (7.1777, -0.4722) (7.1813, -0.4715) (7.1849, -0.4708) (7.1885, -0.4702) (7.1922, -0.4694) (7.1958, -0.4687) (7.1995, -0.468) (7.2033, -0.4673) (7.207, -0.4665) (7.2108, -0.4657) (7.2145, -0.465) (7.2183, -0.4642) (7.2222, -0.4634) (7.226, -0.4625) (7.2299, -0.4617) (7.2338, -0.4609) (7.2377, -0.46) (7.2416, -0.4591) (7.2456, -0.4583) (7.2496, -0.4574) (7.2536, -0.4565) (7.2576, -0.4555) (7.2616, -0.4546) (7.2657, -0.4537) (7.2698, -0.4527) (7.2739, -0.4517) (7.278, -0.4507) (7.2822, -0.4497) (7.2863, -0.4487) (7.2905, -0.4477) (7.2947, -0.4466) (7.299, -0.4456) (7.3032, -0.4445) (7.3075, -0.4434) (7.3118, -0.4423) (7.3161, -0.4412) (7.3204, -0.4401) (7.3247, -0.439) (7.3291, -0.4378) (7.3335, -0.4366) (7.3379, -0.4354) (7.3423, -0.4342) (7.3468, -0.433) (7.3512, -0.4318) (7.3557, -0.4306) (7.3602, -0.4293) (7.3647, -0.428) (7.3692, -0.4267) (7.3738, -0.4254) (7.3784, -0.4241) (7.383, -0.4228) (7.3876, -0.4215) (7.3922, -0.4201) (7.3968, -0.4187) (7.4015, -0.4173) (7.4062, -0.4159) (7.4109, -0.4145) (7.4156, -0.4131) (7.4203, -0.4116) (7.4251, -0.4101) (7.4298, -0.4087) (7.4346, -0.4072) (7.4394, -0.4056) (7.4442, -0.4041) (7.4491, -0.4026) (7.4539, -0.401) (7.4588, -0.3994) (7.4637, -0.3978) (7.4686, -0.3962) (7.4735, -0.3946) (7.4784, -0.393) (7.4834, -0.3913) (7.4884, -0.3896) (7.4933, -0.388) (7.4983, -0.3863) (7.5033, -0.3845) (7.5084, -0.3828) (7.5134, -0.3811) (7.5185, -0.3793) (7.5236, -0.3775) (7.5287, -0.3757) (7.5338, -0.3739) (7.5389, -0.3721) (7.544, -0.3702) (7.5492, -0.3683) (7.5544, -0.3665) (7.5595, -0.3646) (7.5647, -0.3626) (7.5699, -0.3607) (7.5752, -0.3588) (7.5804, -0.3568) (7.5857, -0.3548) (7.591, -0.3528) (7.5962, -0.3508) (7.6015, -0.3488) (7.6069, -0.3467) (7.6122, -0.3447) (7.6175, -0.3426) (7.6229, -0.3405) (7.6283, -0.3384) (7.6336, -0.3362) (7.639, -0.3341) (7.6444, -0.3319) (7.6499, -0.3297) (7.6553, -0.3275) (7.6608, -0.3253) (7.6662, -0.3231) (7.6717, -0.3208) (7.6772, -0.3186) (7.6827, -0.3163) (7.6882, -0.314) (7.6938, -0.3117) (7.6993, -0.3093) (7.7049, -0.307) (7.7104, -0.3046) (7.716, -0.3022) (7.7216, -0.2998) (7.7272, -0.2974) (7.7328, -0.2949) (7.7385, -0.2925) (7.7441, -0.29) (7.7498, -0.2875) (7.7554, -0.285) (7.7611, -0.2824) (7.7668, -0.2799) (7.7725, -0.2773) (7.7782, -0.2747) (7.7839, -0.2721) (7.7885, -0.27) (7.792, -0.2685) (7.7943, -0.2674) (7.7954, -0.2669) knots 0 0 0 0 0 0 0.00416667 0.00833333 0.0125 0.01666667 0.02083333 0.025 0.02916667 0.03333333 0.0375 0.04166667 0.04583333 0.05 0.05416667 0.05833333 0.0625 0.06666667 0.07083333 0.075 0.07916667 0.08333333 0.0875 0.09166667 0.09583333 0.1 0.10416667 0.10833333 0.1125 0.11666667 0.12083333 0.125 0.12916667 0.13333333 0.1375 0.14166667 0.14583333 0.15 0.15416667 0.15833333 0.1625 0.16666667 0.17083333 0.175 0.17916667 0.18333333 0.1875 0.19166667 0.19583333 0.2 0.20416667 0.20833333 0.2125 0.21666667 0.22083333 0.225 0.22916667 0.23333333 0.2375 0.24166667 0.24583333 0.25 0.25416667 0.25833333 0.2625 0.26666667 0.27083333 0.275 0.27916667 0.28333333 0.2875 0.29166667 0.29583333 0.3 0.30416667 0.30833333 0.3125 0.31666667 0.32083333 0.325 0.32916667 0.33333333 0.3375 0.34166667 0.34583333 0.35 0.35416667 0.35833333 0.3625 0.36666667 0.37083333 0.375 0.37916667 0.38333333 0.3875 0.39166667 0.39583333 0.4 0.40416667 0.40833333 0.4125 0.41666667 0.42083333 0.425 0.42916667 0.43333333 0.4375 0.44166667 0.44583333 0.45 0.45416667 0.45833333 0.4625 0.46666667 0.47083333 0.475 0.47916667 0.48333333 0.4875 0.49166667 0.49583333 0.5 0.50416667 0.50833333 0.5125 0.51666667 0.52083333 0.525 0.52916667 0.53333333 0.5375 0.54166667 0.54583333 0.55 0.55416667 0.55833333 0.5625 0.56666667 0.57083333 0.575 0.57916667 0.58333333 0.5875 0.59166667 0.59583333 0.6 0.60416667 0.60833333 0.6125 0.61666667 0.62083333 0.625 0.62916667 0.63333333 0.6375 0.64166667 0.64583333 0.65 0.65416667 0.65833333 0.6625 0.66666667 0.67083333 0.675 0.67916667 0.68333333 0.6875 0.69166667 0.69583333 0.7 0.70416667 0.70833333 0.7125 0.71666667 0.72083333 0.725 0.72916667 0.73333333 0.7375 0.74166667 0.74583333 0.75 0.75416667 0.75833333 0.7625 0.76666667 0.77083333 0.775 0.77916667 0.78333333 0.7875 0.79166667 0.79583333 0.8 0.80416667 0.80833333 0.8125 0.81666667 0.82083333 0.825 0.82916667 0.83333333 0.8375 0.84166667 0.84583333 0.85 0.85416667 0.85833333 0.8625 0.86666667 0.87083333 0.875 0.87916667 0.88333333 0.8875 0.89166667 0.89583333 0.9 0.90416667 0.90833333 0.9125 0.91666667 0.92083333 0.925 0.92916667 0.93333333 0.9375 0.94166667 0.94583333 0.95 0.95416667 0.95833333 0.9625 0.96666667 0.97083333 0.975 0.97916667 0.98333333 0.9875 0.99166667 0.99583333 1 1 1 1 1 1
  spline S1 degree 5 poles (6.9535, 0.4945) (6.9535, 0.4945) (6.9536, 0.4945) (6.9537, 0.4945) (6.9539, 0.4945) (6.9541, 0.4945) (6.9545, 0.4945) (6.9548, 0.4946) (6.9552, 0.4946) (6.9556, 0.4946) (6.9561, 0.4946) (6.9566, 0.4946) (6.9571, 0.4947) (6.9577, 0.4947) (6.9583, 0.4947) (6.959, 0.4947) (6.9597, 0.4947) (6.9604, 0.4948) (6.9611, 0.4948) (6.9619, 0.4948) (6.9628, 0.4948) (6.9636, 0.4948) (6.9646, 0.4948) (6.9655, 0.4949) (6.9665, 0.4949) (6.9675, 0.4949) (6.9685, 0.4949) (6.9696, 0.4949) (6.9707, 0.4949) (6.9719, 0.4949) (6.9731, 0.4949) (6.9743, 0.4949) (6.9756, 0.4949) (6.9769, 0.4948) (6.9782, 0.4948) (6.9796, 0.4948) (6.9809, 0.4948) (6.9824, 0.4948) (6.9838, 0.4947) (6.9853, 0.4947) (6.9869, 0.4946) (6.9884, 0.4946) (6.99, 0.4946) (6.9916, 0.4945) (6.9933, 0.4944) (6.995, 0.4944) (6.9967, 0.4943) (6.9985, 0.4942) (7.0002, 0.4942) (7.0021, 0.4941) (7.0039, 0.494) (7.0058, 0.4939) (7.0077, 0.4938) (7.0096, 0.4937) (7.0116, 0.4936) (7.0136, 0.4934) (7.0156, 0.4933) (7.0177, 0.4932) (7.0198, 0.493) (7.0219, 0.4929) (7.0241, 0.4927) (7.0263, 0.4926) (7.0285, 0.4924) (7.0307, 0.4922) (7.033, 0.4921) (7.0353, 0.4919) (7.0376, 0.4917) (7.04, 0.4915) (7.0424, 0.4913) (7.0448, 0.4911) (7.0472, 0.4908) (7.0497, 0.4906) (7.0522, 0.4903) (7.0548, 0.4901) (7.0573, 0.4898) (7.0599, 0.4896) (7.0625, 0.4893) (7.0652, 0.489) (7.0678, 0.4887) (7.0705, 0.4884) (7.0733, 0.4881) (7.076, 0.4878) (7.0788, 0.4874) (7.0816, 0.4871) (7.0844, 0.4868) (7.0873, 0.4864) (7.0902, 0.486) (7.0931, 0.4857) (7.096, 0.4853) (7.099, 0.4849) (7.102, 0.4845) (7.105, 0.4841) (7.1081, 0.4836) (7.1111, 0.4832) (7.1142, 0.4827) (7.1173, 0.4823) (7.1205, 0.4818) (7.1237, 0.4813) (7.1268, 0.4809) (7.1301, 0.4804) (7.1333, 0.4798) (7.1366, 0.4793) (7.1399, 0.4788) (7.1432, 0.4782) (7.1465, 0.4777) (7.1499, 0.4771) (7.1533, 0.4766) (7.1567, 0.476) (7.1602, 0.4754) (7.1636, 0.4748) (7.1671, 0.4741) (7.1706, 0.4735) (7.1741, 0.4729) (7.1777, 0.4722) (7.1813, 0.4715) (7.1849, 0.4708) (7.1885, 0.4702) (7.1922, 0.4694) (7.1958, 0.4687) (7.1995, 0.468) (7.2033, 0.4673) (7.207, 0.4665) (7.2108, 0.4657) (7.2145, 0.465) (7.2183, 0.4642) (7.2222, 0.4634) (7.226, 0.4625) (7.2299, 0.4617) (7.2338, 0.4609) (7.2377, 0.46) (7.2416, 0.4591) (7.2456, 0.4583) (7.2496, 0.4574) (7.2536, 0.4565) (7.2576, 0.4555) (7.2616, 0.4546) (7.2657, 0.4537) (7.2698, 0.4527) (7.2739, 0.4517) (7.278, 0.4507) (7.2822, 0.4497) (7.2863, 0.4487) (7.2905, 0.4477) (7.2947, 0.4466) (7.299, 0.4456) (7.3032, 0.4445) (7.3075, 0.4434) (7.3118, 0.4423) (7.3161, 0.4412) (7.3204, 0.4401) (7.3247, 0.439) (7.3291, 0.4378) (7.3335, 0.4366) (7.3379, 0.4354) (7.3423, 0.4342) (7.3468, 0.433) (7.3512, 0.4318) (7.3557, 0.4306) (7.3602, 0.4293) (7.3647, 0.428) (7.3692, 0.4267) (7.3738, 0.4254) (7.3784, 0.4241) (7.383, 0.4228) (7.3876, 0.4215) (7.3922, 0.4201) (7.3968, 0.4187) (7.4015, 0.4173) (7.4062, 0.4159) (7.4109, 0.4145) (7.4156, 0.4131) (7.4203, 0.4116) (7.4251, 0.4101) (7.4298, 0.4087) (7.4346, 0.4072) (7.4394, 0.4056) (7.4442, 0.4041) (7.4491, 0.4026) (7.4539, 0.401) (7.4588, 0.3994) (7.4637, 0.3978) (7.4686, 0.3962) (7.4735, 0.3946) (7.4784, 0.393) (7.4834, 0.3913) (7.4884, 0.3896) (7.4933, 0.388) (7.4983, 0.3863) (7.5033, 0.3845) (7.5084, 0.3828) (7.5134, 0.3811) (7.5185, 0.3793) (7.5236, 0.3775) (7.5287, 0.3757) (7.5338, 0.3739) (7.5389, 0.3721) (7.544, 0.3702) (7.5492, 0.3683) (7.5544, 0.3665) (7.5595, 0.3646) (7.5647, 0.3626) (7.5699, 0.3607) (7.5752, 0.3588) (7.5804, 0.3568) (7.5857, 0.3548) (7.591, 0.3528) (7.5962, 0.3508) (7.6015, 0.3488) (7.6069, 0.3467) (7.6122, 0.3447) (7.6175, 0.3426) (7.6229, 0.3405) (7.6283, 0.3384) (7.6336, 0.3362) (7.639, 0.3341) (7.6444, 0.3319) (7.6499, 0.3297) (7.6553, 0.3275) (7.6608, 0.3253) (7.6662, 0.3231) (7.6717, 0.3208) (7.6772, 0.3186) (7.6827, 0.3163) (7.6882, 0.314) (7.6938, 0.3117) (7.6993, 0.3093) (7.7049, 0.307) (7.7104, 0.3046) (7.716, 0.3022) (7.7216, 0.2998) (7.7272, 0.2974) (7.7328, 0.2949) (7.7385, 0.2925) (7.7441, 0.29) (7.7498, 0.2875) (7.7554, 0.285) (7.7611, 0.2824) (7.7668, 0.2799) (7.7725, 0.2773) (7.7782, 0.2747) (7.7839, 0.2721) (7.7885, 0.27) (7.792, 0.2685) (7.7943, 0.2674) (7.7954, 0.2669) knots 0 0 0 0 0 0 0.00416667 0.00833333 0.0125 0.01666667 0.02083333 0.025 0.02916667 0.03333333 0.0375 0.04166667 0.04583333 0.05 0.05416667 0.05833333 0.0625 0.06666667 0.07083333 0.075 0.07916667 0.08333333 0.0875 0.09166667 0.09583333 0.1 0.10416667 0.10833333 0.1125 0.11666667 0.12083333 0.125 0.12916667 0.13333333 0.1375 0.14166667 0.14583333 0.15 0.15416667 0.15833333 0.1625 0.16666667 0.17083333 0.175 0.17916667 0.18333333 0.1875 0.19166667 0.19583333 0.2 0.20416667 0.20833333 0.2125 0.21666667 0.22083333 0.225 0.22916667 0.23333333 0.2375 0.24166667 0.24583333 0.25 0.25416667 0.25833333 0.2625 0.26666667 0.27083333 0.275 0.27916667 0.28333333 0.2875 0.29166667 0.29583333 0.3 0.30416667 0.30833333 0.3125 0.31666667 0.32083333 0.325 0.32916667 0.33333333 0.3375 0.34166667 0.34583333 0.35 0.35416667 0.35833333 0.3625 0.36666667 0.37083333 0.375 0.37916667 0.38333333 0.3875 0.39166667 0.39583333 0.4 0.40416667 0.40833333 0.4125 0.41666667 0.42083333 0.425 0.42916667 0.43333333 0.4375 0.44166667 0.44583333 0.45 0.45416667 0.45833333 0.4625 0.46666667 0.47083333 0.475 0.47916667 0.48333333 0.4875 0.49166667 0.49583333 0.5 0.50416667 0.50833333 0.5125 0.51666667 0.52083333 0.525 0.52916667 0.53333333 0.5375 0.54166667 0.54583333 0.55 0.55416667 0.55833333 0.5625 0.56666667 0.57083333 0.575 0.57916667 0.58333333 0.5875 0.59166667 0.59583333 0.6 0.60416667 0.60833333 0.6125 0.61666667 0.62083333 0.625 0.62916667 0.63333333 0.6375 0.64166667 0.64583333 0.65 0.65416667 0.65833333 0.6625 0.66666667 0.67083333 0.675 0.67916667 0.68333333 0.6875 0.69166667 0.69583333 0.7 0.70416667 0.70833333 0.7125 0.71666667 0.72083333 0.725 0.72916667 0.73333333 0.7375 0.74166667 0.74583333 0.75 0.75416667 0.75833333 0.7625 0.76666667 0.77083333 0.775 0.77916667 0.78333333 0.7875 0.79166667 0.79583333 0.8 0.80416667 0.80833333 0.8125 0.81666667 0.82083333 0.825 0.82916667 0.83333333 0.8375 0.84166667 0.84583333 0.85 0.85416667 0.85833333 0.8625 0.86666667 0.87083333 0.875 0.87916667 0.88333333 0.8875 0.89166667 0.89583333 0.9 0.90416667 0.90833333 0.9125 0.91666667 0.92083333 0.925 0.92916667 0.93333333 0.9375 0.94166667 0.94583333 0.95 0.95416667 0.95833333 0.9625 0.96666667 0.97083333 0.975 0.97916667 0.98333333 0.9875 0.99166667 0.99583333 1 1 1 1 1 1
  spline S2 degree 5 poles (6.9531, -0.4945) (6.9531, -0.4945) (6.9531, -0.4945) (6.9532, -0.4945) (6.9532, -0.4945) (6.9533, -0.4945) (6.9534, -0.4945) (6.9534, -0.4945) (6.9535, -0.4945) (6.9535, -0.4945) knots 0 0 0 0 0 0 0.2 0.4 0.6 0.8 1 1 1 1 1 1
  spline S3 degree 5 poles (6.9531, 0.4945) (6.9531, 0.4945) (6.9531, 0.4945) (6.9532, 0.4945) (6.9532, 0.4945) (6.9533, 0.4945) (6.9534, 0.4945) (6.9534, 0.4945) (6.9535, 0.4945) (6.9535, 0.4945) knots 0 0 0 0 0 0 0.2 0.4 0.6 0.8 1 1 1 1 1 1
  line L0 (0, 0) -> (6.9531, -0.4945)
  line L1 (0, 0) -> (6.9531, 0.4945)
  arc A0 (7.7954, -0.2669) -> (7.7954, 0.2669) centre (0, 0) ccw
  point P0 (6.9546, -0.4945)
  point P1 (6.9564, -0.4946)
  point P2 (6.959, -0.4947)
  point P3 (6.9622, -0.4948)
  point P4 (6.9663, -0.4949)
  point P5 (6.971, -0.4949)
  point P6 (6.9765, -0.4948)
  point P7 (6.9827, -0.4947)
  point P8 (6.9897, -0.4946)
  point P9 (6.9974, -0.4943)
  point P10 (7.0058, -0.4939)
  point P11 (7.0149, -0.4934)
  point P12 (7.0248, -0.4927)
  point P13 (7.0353, -0.4919)
  point P14 (7.0467, -0.4909)
  point P15 (7.0587, -0.4897)
  point P16 (7.0714, -0.4883)
  point P17 (7.0848, -0.4867)
  point P18 (7.099, -0.4849)
  point P19 (7.1139, -0.4828)
  point P20 (7.1294, -0.4805)
  point P21 (7.1457, -0.4778)
  point P22 (7.1626, -0.4749)
  point P23 (7.1803, -0.4717)
  point P24 (7.1986, -0.4682)
  point P25 (7.2176, -0.4643)
  point P26 (7.2373, -0.4601)
  point P27 (7.2576, -0.4555)
  point P28 (7.2787, -0.4506)
  point P29 (7.3003, -0.4452)
  point P30 (7.3227, -0.4395)
  point P31 (7.3456, -0.4333)
  point P32 (7.3693, -0.4267)
  point P33 (7.3935, -0.4197)
  point P34 (7.4184, -0.4122)
  point P35 (7.4439, -0.4042)
  point P36 (7.47, -0.3958)
  point P37 (7.4967, -0.3868)
  point P38 (7.524, -0.3773)
  point P39 (7.5519, -0.3673)
  point P40 (7.5804, -0.3568)
  point P41 (7.6095, -0.3457)
  point P42 (7.6391, -0.3341)
  point P43 (7.6693, -0.3218)
  point P44 (7.7, -0.309)
  point P45 (7.7313, -0.2956)
  point P46 (7.7631, -0.2815)
  point P47 (6.9546, 0.4945)
  point P48 (6.9564, 0.4946)
  point P49 (6.959, 0.4947)
  point P50 (6.9622, 0.4948)
  point P51 (6.9663, 0.4949)
  point P52 (6.971, 0.4949)
  point P53 (6.9765, 0.4948)
  point P54 (6.9827, 0.4947)
  point P55 (6.9897, 0.4946)
  point P56 (6.9974, 0.4943)
  point P57 (7.0058, 0.4939)
  point P58 (7.0149, 0.4934)
  point P59 (7.0248, 0.4927)
  point P60 (7.0353, 0.4919)
  point P61 (7.0467, 0.4909)
  point P62 (7.0587, 0.4897)
  point P63 (7.0714, 0.4883)
  point P64 (7.0848, 0.4867)
  point P65 (7.099, 0.4849)
  point P66 (7.1139, 0.4828)
  point P67 (7.1294, 0.4805)
  point P68 (7.1457, 0.4778)
  point P69 (7.1626, 0.4749)
  point P70 (7.1803, 0.4717)
  point P71 (7.1986, 0.4682)
  point P72 (7.2176, 0.4643)
  point P73 (7.2373, 0.4601)
  point P74 (7.2576, 0.4555)
  point P75 (7.2787, 0.4506)
  point P76 (7.3003, 0.4452)
  point P77 (7.3227, 0.4395)
  point P78 (7.3456, 0.4333)
  point P79 (7.3693, 0.4267)
  point P80 (7.3935, 0.4197)
  point P81 (7.4184, 0.4122)
  point P82 (7.4439, 0.4042)
  point P83 (7.47, 0.3958)
  point P84 (7.4967, 0.3868)
  point P85 (7.524, 0.3773)
  point P86 (7.5519, 0.3673)
  point P87 (7.5804, 0.3568)
  point P88 (7.6095, 0.3457)
  point P89 (7.6391, 0.3341)
  point P90 (7.6693, 0.3218)
  point P91 (7.7, 0.309)
  point P92 (7.7313, 0.2956)
  point P93 (7.7631, 0.2815)
sketch "Sketch2" plane through (0, 0, 0) normal (0, 0, 1) x (1, 0, 0)
  circle A0 centre (0, 0) radius 6.45
extrude "Extrude1" add sketch "Sketch2" along normal blind 3 makes body 1